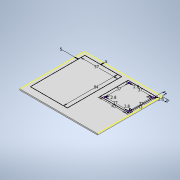
# Autodesk Inventor part: Part1
Saved by Autodesk Inventor 2021.3 (Build 253353010, 353A)
## iProperties
Created: 2021-10-29
Part Number: Part1
Material: Generic
Document SubType Name: Modeling
Designer: jesse
Density: 1 g/cm^3
Appearance: Default
Author: jesse
Autodesk Inventor part; units mm, degrees
ref_plane "YZ Plane" through (0, 0, 0) normal (1, 0, 0) x (0, 1, 0)
ref_plane "XZ Plane" through (0, 0, 0) normal (0, 1, 0) x (-1, 0, 0)
ref_plane "XY Plane" through (0, 0, 0) normal (0, 0, 1) x (1, 0, 0)
sketch "Sketch1" plane through (0, 0, 0) normal (0, 1, 0) x (-1, 0, 0)
  line L0 (4.1192, 94.9482) -> (-115.8808, 94.9482)
  line L1 (-115.8808, 94.9482) -> (-115.8808, -5.0518)
  line L2 (-115.8808, -5.0518) -> (4.1192, -5.0518)
  line L3 (4.1192, -5.0518) -> (4.1192, 94.9482)
  point P0 (0, 0)
  dimension "d0" = 100
  dimension "d1" = 120
  constraints: 8 end point, 2 parallel, 1 horizontal, 1 perpendicular
  measures "d0" distance of L2.end L0.start
  measures "d1" distance of L1.end L2.end
extrude "Extrusion1" add sketch "Sketch1" along normal blind 2
sketch "Sketch2" plane through (0, 2, 0) normal (0, 1, 0) x (1, 0, 0)
  line L0 (0.8808, 0.0518) -> (57.8808, 0.0518)
  line L1 (57.8808, 0.0518) -> (57.8808, -83.9482)
  line L2 (57.8808, -83.9482) -> (0.8808, -83.9482)
  line L3 (0.8808, -83.9482) -> (0.8808, 0.0518)
  line L4 (67.8808, 0.0518) -> (110.8808, 0.0518)
  line L5 (110.8808, 0.0518) -> (110.8808, -42.9482)
  line L6 (110.8808, -42.9482) -> (67.8808, -42.9482)
  line L7 (67.8808, -42.9482) -> (67.8808, 0.0518)
  line L8 (115.8808, 5.0518) -> (-4.1192, 5.0518) projected
  line L9 (115.8808, -94.9482) -> (115.8808, 5.0518) projected
  line L10 (-4.1192, 5.0518) -> (-4.1192, -94.9482) projected
  circle A0 centre (72.2653, -2.7404) radius 1.4
  circle A1 centre (109.2543, -3.6401) radius 1.4
  circle A2 centre (109.7111, -40.6373) radius 1.4
  circle A3 centre (72.722, -39.7376) radius 1.4
  point P0 (0, 0)
  dimension "d4" = 57
  dimension "d5" = 84
  dimension "d6" = 43
  dimension "d7" = 43
  dimension "d8" = 5
  dimension "d9" = 5
  dimension "d10" = 5
  dimension "d11" = 5
  dimension "d12" = 2.8
  dimension "d13" = 2.8
  dimension "d14" = 2.8
  dimension "d15" = 2.8
  dimension "d16" = 37
  dimension "d17" = 37
  dimension "d18" = 37
  dimension "d19" = 37
  constraints: 16 end point, 4 centre point, 4 parallel, 2 horizontal, 2 perpendicular
  measures "d4" distance of L0.start L0.end
  measures "d5" distance of L0.end L1.end
  measures "d6" distance of L4.end L5.end
  measures "d7" distance of L5.end L6.end
  measures "d8" distance between parallel lines of L8 L4
  measures "d9" distance between parallel lines of L9 L5
  measures "d10" distance between parallel lines of L8 L0
  measures "d11" distance between parallel lines of L10 L3
  measures "d12" diameter of A0
  measures "d13" diameter of A1
  measures "d14" diameter of A2
  measures "d15" diameter of A3
  measures "d16" distance of A1.centre A0.centre
  measures "d17" distance of A2.centre A3.centre
  measures "d18" distance of A2.centre A1.centre
  measures "d19" distance of A3.centre A0.centre
body "Solid1"
